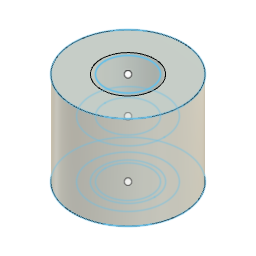
pillar (Autodesk Fusion 360 design; units mm, degrees)
Autodesk Fusion 360 part; units mm, degrees
sketch "sketch 714" plane through (0, 0, 0.8823) normal (0, 0, -1) x (1, 0, 0)
  circle A0 centre (235.6841, 105.0114) radius 1.2645
  circle A1 centre (235.6841, 105.0114) radius 3
extrude "拉伸1" add sketch "sketch 714" along normal blind 2
sketch "sketch 730" plane through (0, 0, -1.1177) normal (0, 0, -1) x (1, 0, 0)
  circle A0 centre (235.6841, 105.0114) radius 1.2645
  circle A1 centre (235.6841, 105.0114) radius 2
extrude "拉伸2" add sketch "sketch 730" along normal blind 3.12
sketch "sketch 745" plane through (0, 0, -4.2377) normal (0, 0, -1) x (1, 0, 0)
  circle A0 centre (235.6841, 105.0114) radius 1.2645
  circle A1 centre (235.6841, 105.0114) radius 1.4645
extrude "拉伸3" cut sketch "sketch 745" against normal up to surface (5.12 mm away)
sketch "sketch 760" plane through (0, 0, -4.2377) normal (0, 0, -1) x (1, 0, 0)
  circle A0 centre (235.6841, 105.0114) radius 2
  circle A1 centre (235.6841, 105.0114) radius 3
extrude "拉伸4" add sketch "sketch 760" against normal blind 2
extrude "拉伸5" add 1 faces at (233.1905, -104.0863, -2.2377) along direction (0, 0, 1) blind 1.12
